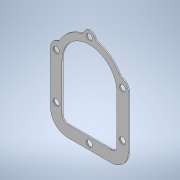
# Autodesk Inventor part: 411. Прокладка
Saved by Autodesk Inventor 2021 (Build 250183000, 183)
## iProperties
Created: 2021-04-18
Part Number: 411. Прокладка
Material: Типовые
Document SubType Name: Modeling
Designer: Данил
Density: 1 g/cm^3
Appearance: По умолчанию
Author: Данил
Autodesk Inventor part; units mm, degrees
ref_plane "YZ Plane" through (0, 0, 0) normal (1, 0, 0) x (0, 1, 0)
ref_plane "XZ Plane" through (0, 0, 0) normal (0, 1, 0) x (-1, 0, 0)
ref_plane "XY Plane" through (0, 0, 0) normal (0, 0, 1) x (1, 0, 0)
sketch "Эскиз1" plane through (0, 0, 0) normal (0, 0, 1) x (1, 0, 0)
  line L0 (-48.5, 29) -> (-48.5, -54)
  line L1 (-38.5, -64) -> (38.5, -64)
  line L2 (48.5, -54) -> (48.5, 29)
  arc A0 (38.5, -64) -> (48.5, -54) centre (38.5, -54) ccw
  arc A1 (-48.5, -54) -> (-38.5, -64) centre (-38.5, -54) ccw
  line L3 (-38.5, -84) -> (38.5, -84)
  line L4 (68.5, -54) -> (68.5, 40)
  line L5 (-68.5, -54) -> (-68.5, 40)
  circle A2 centre (0, -74) radius 5.25
  circle A3 centre (-58.5, -40) radius 5.25
  circle A4 centre (58.5, -40) radius 5.25
  arc A5 (-57.7881, 54.374) -> (-68.5, 40) centre (-53.5, 40) ccw
  arc A6 (-57.7881, 54.374) -> (-51.9829, 58.9629) centre (-60.6468, 63.9567) ccw
  arc A7 (-15.8919, 86.8571) -> (-51.9829, 58.9629) centre (0, 29) ccw
  arc A8 (-15.8919, 86.8571) -> (-9.2702, 92.75) centre (-18.5405, 96.5) ccw
  arc A9 (9.2702, 92.75) -> (-9.2702, 92.75) centre (0, 89) ccw
  circle A10 centre (-58.5, 40) radius 5.25
  arc A11 (9.2702, 92.75) -> (15.8919, 86.8571) centre (18.5405, 96.5) ccw
  arc A12 (51.9829, 58.9629) -> (15.8919, 86.8571) centre (0, 29) ccw
  arc A13 (51.9829, 58.9629) -> (57.7881, 54.374) centre (60.6468, 63.9567) ccw
  arc A14 (68.5, 40) -> (57.7881, 54.374) centre (53.5, 40) ccw
  circle A15 centre (58.5, 40) radius 5.25
  circle A16 centre (0, 89) radius 5.25
  arc A17 (38.5, -84) -> (68.5, -54) centre (38.5, -54) ccw
  arc A18 (-68.5, -54) -> (-38.5, -84) centre (-38.5, -54) ccw
  arc A19 (48.5, 29) -> (-48.5, 29) centre (0, 29) ccw
  point P0 (0, 0)
  point P1 (-48.5, -64)
  point P2 (48.5, -64)
  point P3 (0, -64)
  dimension "d0" = 97
  dimension "d1" = 10
  dimension "d2" = 20
  dimension "d3" = 20
  dimension "d4" = 20
  dimension "d5" = 10.5
  dimension "d6" = 10
  dimension "d7" = 74
  dimension "d8" = 58.5
  dimension "d9" = 58.5
  dimension "d10" = 15
  dimension "d11" = 10
  dimension "d12" = 60
  dimension "d13" = 29
  dimension "d14" = 10
  dimension "d15" = 40
  dimension "d16" = 80
  dimension "d17" = 30
  dimension "d18" = 163
  constraints: 28 point on circle, 20 centre point, 19 tangent, 12 end point, 12 equal radius, 8 vertical alignment, 5 horizontal alignment, 4 point on line, 3 coincident, 3 perpendicular, 2 vertical, 1 horizontal, 1 midpoint
  measures "d0" distance of point (-48.5, -64) point (48.5, -64)
  measures "d1" radius of A0
  measures "d2" distance between parallel lines of L3 L1
  measures "d3" distance between parallel lines of L4 L2
  measures "d4" distance between parallel lines of L5 L0
  measures "d5" diameter of A2
  measures "d6" distance of point (0, -64) A2.centre
  measures "d7" distance of point (0, 0) A2.centre
  measures "d8" horizontal distance of A4.centre point (0, 0)
  measures "d9" horizontal distance of point (0, 0) A3.centre
  measures "d10" radius of A5
  measures "d11" radius of A6
  measures "d12" radius of A7
  measures "d13" distance of A7.centre point (0, 0)
  measures "d14" radius of A9
  measures "d15" vertical distance of point (0, 0) A15.centre
  measures "d16" distance of A3.centre A10.centre
  measures "d17" radius of A17
  measures "d18" distance of A2.centre A9.centre
extrude "Выдавливание1" add sketch "Эскиз1" along normal mid plane 2
